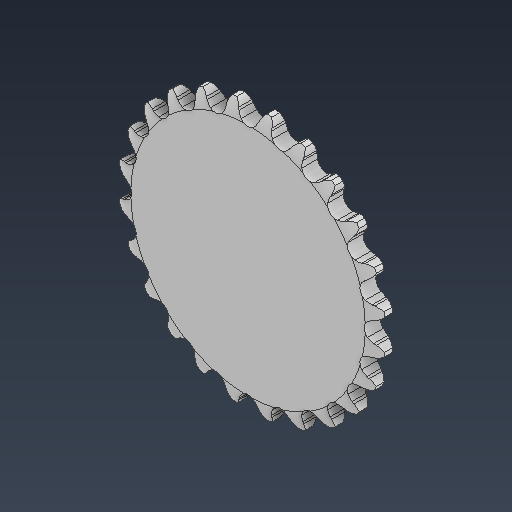
# Autodesk Inventor part: Звездочка роликовой цепи1
Saved by Autodesk Inventor 2025 (Build 290162000, 162)
## iProperties
CustomPartVersion: 1
Created: 2024-09-18
Part Number: Звездочка роликовой цепи1
Material: Пластик ПЭТ
Document SubType Name: Modeling
Designer: GameHD
Density: 1.541 g/cm^3
Appearance: Поликарбонат — прозрачный
d28: 0,000 мм
d29: 0,000 мм
d42: 0,000 мм
Author: GameHD
Autodesk Inventor part; units mm, degrees
ref_plane "YZ Plane" through (0, 0, 0) normal (1, 0, 0) x (0, 1, 0)
ref_plane "XZ Plane" through (0, 0, 0) normal (0, 1, 0) x (-1, 0, 0)
ref_plane "XY Plane" through (0, 0, 0) normal (0, 0, 1) x (1, 0, 0)
sketch "Теоретический профиль зуба" plane through (0, 0, 0) normal (0, 0, 1) x (1, 0, 0)
  circle A0 centre (0, 0) radius 24.3246 construction
  line L0 (0, 0) -> (0, 24.3246) construction
  line L1 (0, 0) -> (6.2957, 23.4958) construction
  circle A1 centre (0, 0) radius 26.0215
  arc A2 (-1.3466, 23.2913) -> (1.3466, 23.2913) centre (0, 24.3246) ccw
  line L2 (0, 24.3246) -> (6.2957, 23.4958) construction
  line L3 (0, 24.3246) -> (2.0957, 25.9327) construction
  line L4 (2.0957, 25.9327) -> (-1.932, 24.319) construction
  arc A3 (2.9539, 25.8533) -> (2.0923, 24.7192) centre (4.5833, 23.7212) ccw
  arc A4 (-2.0923, 24.7192) -> (-2.9539, 25.8533) centre (-4.5833, 23.7212) ccw
  line L5 (-4.5833, 23.7212) -> (-2.0923, 24.7192) construction
  arc A5 (-1.932, 24.319) -> (-1.3466, 23.2913) centre (2.0957, 25.9327) ccw
  line L6 (-1.932, 24.319) -> (-2.0923, 24.7192)
  arc A6 (1.3466, 23.2913) -> (1.932, 24.319) centre (-2.0957, 25.9327) ccw
  line L7 (2.0923, 24.7192) -> (1.932, 24.319)
  line L8 (0, 0) -> (3.3965, 25.7989) construction
  point P0 (3.1478, 23.9102)
  dimension "d0" = 48.6492
  dimension "d2" = 15
  dimension "d3" = 1.6974
  dimension "d10" = 127.5
  dimension "d11" = 15.667
  dimension "d12" = 2.6416
  dimension "d13" = 4.339
  dimension "d14" = 4.6228
  dimension "d23" = 1.905
  constraints: 18 end point, 15 point on circle, 7 centre point, 3 coincident, 3 point on line, 3 symmetric about line, 3 tangent, 1 equal radius, 1 midpoint, 1 parallel, 1 vertical, 1 other
  measures "d0" diameter of A0
  measures "d2" angle of L1 L0
  measures "d3" radius of A2
  measures "d10" angle of L3 L0
  measures "d11" angle of L4 L3
  measures "d12" distance of L2.start L3.end
  measures "d13" distance of L3.end L4.end
  measures "d14" distance of A3.centre L0.end
  measures "d23" distance from line of L8.end L2
sketch "Профиль зуба" plane through (0, 0, 0) normal (0, 0, 1) x (1, 0, 0)
  arc A0 (-1.5751, 23.6922) -> (1.5751, 23.6922) centre (0, 24.3246) ccw
  arc A1 (2.7748, 25.8732) -> (1.5751, 23.6922) centre (11.1356, 19.8538) ccw
  arc A2 (-1.5751, 23.6922) -> (-2.7748, 25.8732) centre (-11.1356, 19.8538) ccw
  line L0 (0, 0) -> (0, 24.3246) construction
  line L1 (0, 24.3246) -> (1.5751, 23.6922) construction
  line L2 (0, 24.3246) -> (-1.5751, 23.6922) construction
  circle A3 centre (0, 0) radius 26.0215 projected
  dimension "d44" = 136.25
  dimension "d45" = 10.3022
  dimension "d46" = 1.6974
  constraints: 9 point on circle, 6 end point, 3 centre point, 2 tangent, 1 coincident, 1 equal radius, 1 vertical, 1 other
  measures "d44" angle of L2 L1
  measures "d45" radius of A1
  measures "d46" radius of A0
sketch "Профиль сечения" plane through (0, 0, 0) normal (1, 0, 0) x (0, 1, 0)
  line L0 (26.0215, 0) -> (-26.0215, 0) projected
  line L1 (20.3065, 1.5526) -> (-20.3065, 1.5526)
  line L2 (-20.3065, 1.5526) -> (-20.3065, -1.5526)
  line L3 (-20.3065, -1.5526) -> (20.3065, -1.5526)
  line L4 (20.3065, -1.5526) -> (20.3065, 1.5526)
  line L5 (20.3065, 1.5526) -> (26.0215, 1.5526) construction
  line L6 (26.0215, 1.5526) -> (26.0215, -1.5526) construction
  line L7 (26.0215, -1.5526) -> (20.3065, -1.5526) construction
  line L8 (20.3065, -1.5526) -> (20.3065, 1.5526)
  arc A0 (26.0215, 0.7588) -> (22.8457, 1.5526) centre (22.8457, -5.1975) ccw
  arc A1 (22.8457, -1.5526) -> (26.0215, -0.7588) centre (22.8457, 5.1975) ccw
  line L9 (22.8457, 1.5526) -> (0, 1.5526)
  line L10 (0, 1.5526) -> (0, -1.5526)
  line L11 (0, -1.5526) -> (22.8457, -1.5526)
  line L12 (0, 1.5526) -> (0, -1.5526)
  line L13 (26.0215, 0.7588) -> (26.0215, -0.7588)
  point P0 (0, 0)
  point P1 (0, 0)
  dimension "d30" = 3.1052
  dimension "d31" = 40.613
  dimension "d32" = 3.1052
  dimension "d33" = 0.7937
  dimension "d34" = 6.75
  dimension "d43" = 1.5526
  constraints: 26 end point, 7 midpoint, 5 perpendicular, 4 parallel, 4 point on circle, 3 point on line, 3 symmetric about line, 2 centre point, 2 horizontal, 2 tangent, 1 collinear, 1 other
  measures "d30" distance between parallel lines of L7 L5
  measures "d31" distance between parallel lines of L2 L4
  measures "d32" distance between parallel lines of L3 L1
  measures "d33" distance from line of L13.start L5
  measures "d34" radius of A0
  measures "d43" distance between parallel lines of L3 L0
revolve "Диск" add sketch "Профиль сечения" angle 360 about axis through (0, 0, 1.5526) along (0, 0, -1) contours L10 L3 L2 L0 | L0 L2 L1 L10
revolve "Ветвь" add sketch "Профиль сечения" angle 360 about axis through (0, 0, 1.5526) along (0, 0, -1) contours L13 A1 L11 L4 L0 | L0 L4 L9 A0 L13 | L4 L3 L10 L0 | L0 L10 L1 L4
fillet "Fillet2" [suppressed]
pattern_of_one "Массив ветвей"
extrude "Теоретический зуб" cut sketch "Теоретический профиль зуба" along normal through all both and the other way through all contours A3 L7 A6 A2 A5 L6 A4 A1 picked at (0.3288, 24.4113)
extrude "Зуб" [suppressed]
pattern_circular "Форма зуба" count 24 over 360 about axis through (0, 0, -10) along (0, 0, 1) of "Теоретический зуб"
ref_plane "Плоскость синхронизации" through (0, 24.3246, 0) normal (1, 0, 0) x (0, 1, 0)
equation "\"d3\" = 0.5 * da_Dr + da_SC"
equation "\"d12\" = 0.8 * da_Dr"
equation "\"d13\" = 1.3 * da_Dr + da_SC"
equation "\"d14\" = 1.4 * da_Dr"
equation "\"d23\" = da_Ha"
equation "\"d44\" = da_Alfa"
equation "\"d45\" = da_Re"
equation "\"d46\" = da_Ri"
equation "\"d30\" = da_Bf"
equation "\"d31\" = da_Ds"
equation "\"d32\" = da_Bs"
equation "\"d33\" = da_Ba"
equation "\"d34\" = da_Rx"
equation "\"d51\" = da_Ra"
equation "\"d40\" = da_pt"
equation "\"form_type\" = 0"
equation "\"da_p\" = 6.35"
equation "\"da_Dr\" = 3.302"
equation "\"da_SC\" = 0.04636"
equation "\"da_Ha\" = 1.905"
equation "\"da_pt\" = 6.4008"
equation "\"da_Bf\" = 3.10515"
equation "\"da_Ba\" = 0.79375"
equation "\"da_Rx\" = 6.75005"
equation "\"da_Ra\" = 0.254"
equation "\"da_Bs\" = 3.10515"
equation "\"da_Ds\" = 40.61304"
equation "\"da_Re\" = 10.30224"
equation "\"da_Ri\" = 1.69736"
equation "\"da_Alfa\" = 136.25deg"
body "Solid1"
